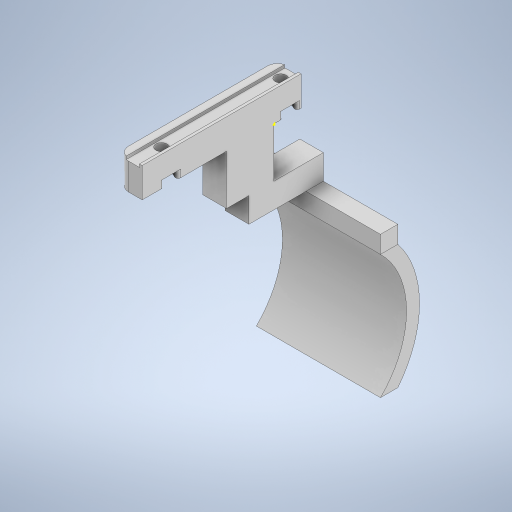
# Autodesk Inventor part: Back
Saved by Autodesk Inventor 2024 (Build 280153000, 153)
## iProperties
Created: 2023-12-18
Part Number: Back
Material: Generic
Document SubType Name: Modeling
Designer: Mechatronics Lab 1
Density: 1 g/cm^3
Appearance: Default
Author: Mechatronics Lab 1
Autodesk Inventor part; units mm, degrees
ref_plane "YZ Plane" through (0, 0, 0) normal (1, 0, 0) x (0, 1, 0)
ref_plane "XZ Plane" through (0, 0, 0) normal (0, 1, 0) x (-1, 0, 0)
ref_plane "XY Plane" through (0, 0, 0) normal (0, 0, 1) x (1, 0, 0)
sketch "Sketch1" plane through (0, 0, 0) normal (0, 1, 0) x (-1, 0, 0)
  line L0 (0, 0) -> (9.5, 0)
  line L1 (9.5, 0) -> (9.5, -64)
  line L2 (9.5, -64) -> (0, -64)
  line L3 (0, -64) -> (0, 0)
  circle A0 centre (3.7, -11.5) radius 2.25
  circle A1 centre (3.7, -59.5) radius 2.25
  line L4 (3.7, -11.5) -> (3.7, -59.5) construction
  dimension "d1" = 9.5
  dimension "d2" = 64
  dimension "d3" = 4.5
  dimension "d4" = 48
  dimension "d6" = 3.7
  dimension "d17" = 4.5
  constraints: 10 end point, 2 centre point, 2 parallel, 1 equal radius, 1 horizontal, 1 perpendicular, 1 vertical
  measures "d1" distance of L0.start L0.end
  measures "d2" distance of L0.end L1.end
  measures "d3" diameter of A0
  measures "d4" distance of L4.start L4.end
  measures "d6" distance between parallel lines of L3 L4
  measures "d17" distance from line of L4.end L2
extrude "Extrusion1" add sketch "Sketch1" along normal blind 12
sketch "Sketch2" plane through (-9.5, 0, 0) normal (0, 0, 1) x (1, 0, 0)
  line L0 (9.5, 12) -> (0, 12) projected
  line L1 (3, 12) -> (8.4, 12)
  line L2 (8.4, 12) -> (8.4, 10.8)
  line L3 (8.4, 10.8) -> (3, 10.8)
  line L4 (3, 10.8) -> (3, 12)
  line L5 (9.5, 0) -> (9.5, 12) projected
  line L6 (3.55, 0) -> (8.05, 0) projected
  line L7 (3.55, 12) -> (8.05, 12) projected
  line L8 (9.5, 0) -> (9.5, 12) projected
  line L9 (9.5, 0) -> (9.5, 12) projected
  line L10 (3.55, 12) -> (8.05, 12) projected
  line L11 (3.55, 12) -> (3.55, 0) projected
  line L12 (3.55, 12) -> (8.05, 12) projected
  line L13 (3.55, 0) -> (8.05, 0) projected
  line L14 (3.55, 12) -> (8.05, 12) projected
  line L15 (3.55, 0) -> (8.05, 0) projected
  line L16 (3.55, 12) -> (8.05, 12) projected
  line L17 (3.55, 0) -> (8.05, 0) projected
  dimension "d9" = 1.1
  dimension "d10" = 5.4
  dimension "d11" = 1.2
  dimension "d76" = 12
  constraints: 8 end point, 2 parallel, 1 horizontal, 1 perpendicular, 1 point on line
  measures "d9" distance between parallel lines of L5 L2
  measures "d10" distance of L2.end L3.end
  measures "d11" distance between parallel lines of L0 L3
  measures "d76" distance between parallel lines of L6 L7
extrude "Extrusion2" cut sketch "Sketch2" against normal up to next
sketch "Sketch3" plane through (0, 0, 0) normal (0, -1, 0) x (1, 0, 0)
  circle A0 centre (-3.7, -11.5) radius 2.25 projected
  circle A1 centre (-3.7, -11.5) radius 3.75
  circle A2 centre (-3.7, -59.5) radius 2.25 projected
  circle A3 centre (-3.7, -59.5) radius 3.75
  point P0 (0, 0)
  dimension "d14" = 7.5
  constraints: 2 centre point, 2 coincident, 1 equal radius
  measures "d14" diameter of A3
extrude "Extrusion3" cut sketch "Sketch3" against normal blind 3
fillet "Fillet1" radius 1 4 edges at (0, 1.5, -58.8897) (0, 1.5, -60.1103) (0, 1.5, -10.8897) (0, 1.5, -12.1103)
fillet "Fillet2" radius 4 2 edges at (-9.5, 6, -64) (-9.5, 6, 0)
sketch "Sketch28" plane through (0, 0, 0) normal (0, -1, 0) x (1, 0, 0)
  arc A0 (-1.5684, -56.4147) -> (0, -55.592) centre (-1, -55.592) ccw projected
  line L0 (0, -55.592) -> (0, -53)
  line L1 (0, -15.408) -> (0, -55.592) projected
  line L2 (-9.5, -60) -> (-9.5, -4) projected
  line L3 (0, -53) -> (-9.5, -53)
  line L4 (-9.5, -53) -> (-9.5, -34)
  line L5 (-9.5, -34) -> (0, -34)
  line L6 (0, -34) -> (0, -53)
  point P0 (0, 0)
  point P1 (0, -34)
  dimension "d107" = 2.592
  dimension "d108" = 19
  constraints: 10 end point, 2 parallel, 2 point on line, 1 horizontal, 1 perpendicular
  measures "d107" distance of L0.start L0.end
  measures "d108" distance of L3.end L4.end
extrude "Extrusion19" add sketch "Sketch28" along normal blind 20
sketch "Sketch40" plane through (0, -20, 0) normal (0, -1, 0) x (1, 0, 0)
  line L0 (0, -53) -> (-9.5, -53) projected
  line L1 (-9.5, -53) -> (-9.5, -73)
  line L2 (-9.5, -73) -> (0, -73)
  line L3 (0, -73) -> (0, -43)
  line L4 (0, 0) -> (0, -64) projected
  line L5 (0, -43) -> (-9.5, -43)
  line L6 (-9.5, -43) -> (-9.5, -53)
  line L7 (-9.5, -43) -> (0, -43)
  line L8 (0, -43) -> (0, -73)
  line L9 (0, -73) -> (-9.5, -73)
  line L10 (-9.5, -73) -> (-9.5, -43)
  dimension "d130" = 20
  dimension "d131" = 30
  constraints: 18 end point, 3 perpendicular, 2 parallel, 2 point on line, 1 collinear, 1 horizontal, 1 vertical
  measures "d130" distance of L0.end L1.end
  measures "d131" distance of L2.end L3.end
extrude "Extrusion21" add sketch "Sketch40" along normal blind 10
sketch "Sketch41" plane through (0, 0, -53) normal (0, 0, -1) x (-1, 0, 0)
  point P0 (0, 0)
sketch "Sketch42" plane through (0, -30, 0) normal (0, -1, 0) x (1, 0, 0)
  line L0 (0, -73) -> (0, -53) projected
  line L1 (0, -73) -> (30, -73)
  line L2 (30, -73) -> (30, -66)
  line L3 (30, -66) -> (-20, -66)
  line L4 (-20, -66) -> (-20, -73)
  line L5 (-20, -73) -> (0, -73)
  point P0 (0, 0)
  dimension "d134" = 30
  dimension "d135" = 7
  dimension "d137" = 50
  constraints: 10 end point, 3 perpendicular, 2 horizontal
  measures "d134" distance of L0.start L1.end
  measures "d135" distance of L1.end L2.end
  measures "d137" distance of L2.end L3.end
extrude "Extrusion22" add sketch "Sketch42" along normal blind 7
sketch "Sketch50" plane through (-20, -30, -73) normal (-1, 0, 0) x (0, 0, 1)
  arc A0 (7, -7) -> (7, -57) centre (31.4949, -32) ccw
  point P0 (73, 30)
  dimension "d147" = 50
  dimension "d148" = 35
  constraints: 2 point on circle, 1 centre point
  measures "d147" distance of A0.start A0.end
  measures "d148" radius of A0
sketch "Sketch51" plane through (0, -37, 0) normal (0, -1, 0) x (1, 0, 0)
  line L0 (-20, -73) -> (30, -73) projected
  line L1 (30, -66) -> (-20, -66) projected
  line L2 (-20, -73) -> (30, -73)
  line L3 (30, -73) -> (30, -66)
  line L4 (30, -66) -> (-20, -66)
  line L5 (-20, -66) -> (-20, -73)
  point P0 (0, 0)
  constraints: 8 end point, 2 parallel, 1 horizontal, 1 perpendicular
sweep "Sweep4" add profiles "Sketch51" path "Sketch50" separate body
sketch "Sketch57" plane through (-20, -37, -73) normal (-1, 0, 0) x (0, 0, 1)
  arc A0 (7, 0) -> (7, -50) centre (31.4949, -25) ccw projected
  line L0 (7, -50) -> (-5.0576, -50)
  line L1 (-5.0576, -50) -> (-5.0576, -59.7183)
  line L2 (-5.0576, -50) -> (16.6451, -50)
  line L3 (16.6451, -50) -> (16.6451, -65.0945)
  line L4 (16.6451, -65.0945) -> (-5.0576, -65.0945)
  line L5 (-5.0576, -65.0945) -> (-5.0576, -50)
  point P0 (73, 37)
  constraints: 12 end point, 2 horizontal, 2 parallel, 2 perpendicular
extrude "Extrusion24" cut sketch "Sketch57" against normal blind 97.95 bodies 2
body "Solid1"
body "Solid2"
